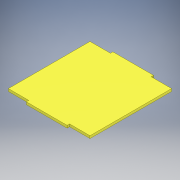
# Autodesk Inventor part: Control lateral
Saved by Autodesk Inventor 2018 (Build 220112000, 112)
## iProperties
Created: 2020-03-09
Part Number: Control lateral
Material: Genérico
Document SubType Name: Modeling
Designer: joser
Density: 1 g/cm^3
Appearance: Suave - Amarillo
Author: joser
Autodesk Inventor part; units mm, degrees
ref_plane "YZ Plane" through (0, 0, 0) normal (1, 0, 0) x (0, 1, 0)
ref_plane "XZ Plane" through (0, 0, 0) normal (0, 1, 0) x (-1, 0, 0)
ref_plane "XY Plane" through (0, 0, 0) normal (0, 0, 1) x (1, 0, 0)
sketch "Boceto1" plane through (0, 0, 0) normal (0, 0, 1) x (1, 0, 0)
  line L0 (0, 100) -> (0, 0)
  line L1 (-75, 0) -> (-75, -3)
  line L2 (-75, -3) -> (-25, -3)
  line L3 (-25, -3) -> (-25, 0)
  line L4 (0, 0) -> (-25, 0)
  line L5 (-100, 0) -> (-75, 0)
  line L6 (-75, 100) -> (-75, 103)
  line L7 (-75, 103) -> (-25, 103)
  line L8 (-25, 103) -> (-25, 100)
  line L9 (0, 100) -> (-25, 100)
  line L10 (-75, 100) -> (-100, 100)
  line L11 (-100, 100) -> (-100, 0)
  dimension "d1" = 100
  dimension "d4" = 50
  dimension "d5" = 25
  dimension "d10" = 3
  dimension "d13" = 50
  dimension "d14" = 3
  dimension "d37" = 100
  constraints: 24 end point, 5 perpendicular, 3 collinear, 3 horizontal, 3 vertical, 1 coincident
  measures "d1" distance of L0.start L0.end
  measures "d4" distance of L1.end L2.end
  measures "d5" distance between parallel lines of L0 L3
  measures "d10" distance between parallel lines of L5 L2
  measures "d13" distance of L6.end L7.end
  measures "d14" distance between parallel lines of L10 L7
  measures "d37" distance between parallel lines of L0 L11
extrude "Extrusión2" add sketch "Boceto1" along normal blind 3
